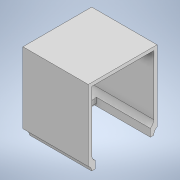
# Autodesk Inventor part: NEMA17_Shroud
Saved by Autodesk Inventor 2021 (Build 250183000, 183)
## iProperties
Created: 2021-10-06
Part Number: NEMA17_Shroud
Material: Generic
Document SubType Name: Modeling
Designer: Jorian Brusind
Density: 1 g/cm^3
Appearance: Default
Author: Jorian Brusind
Autodesk Inventor part; units mm, degrees
ref_plane "YZ Plane" through (0, 0, 0) normal (1, 0, 0) x (0, 1, 0)
ref_plane "XZ Plane" through (0, 0, 0) normal (0, 1, 0) x (-1, 0, 0)
ref_plane "XY Plane" through (0, 0, 0) normal (0, 0, 1) x (1, 0, 0)
sketch "Sketch1" plane through (0, 0, 0) normal (0, 1, 0) x (-1, 0, 0)
  line L0 (0, 0) -> (55, 0)
  line L1 (55, 0) -> (55, -55)
  line L2 (55, -55) -> (0, -55)
  line L3 (0, -58) -> (58, -58)
  line L4 (58, -58) -> (58, 3)
  line L5 (58, 3) -> (0, 3)
  line L6 (0, 3) -> (0, 0)
  line L7 (0, -55) -> (0, -58)
  dimension "d0" = 55
  dimension "d1" = 55
  dimension "d2" = 3
  constraints: 16 end point, 3 equal length, 2 perpendicular, 1 horizontal, 1 vertical, 2 other
  measures "d0" distance of L1.end L2.end
  measures "d1" distance of L0.end L1.end
  measures "d2" distance between parallel lines of L1 L4
extrude "Extrusion1" add sketch "Sketch1" along normal blind 60
sketch "Sketch2" plane through (0, 60, 0) normal (0, 1, 0) x (1, 0, 0)
  line L0 (-58, 58) -> (-58, -3) projected
  line L1 (0, 55) -> (0, 58) projected
  line L2 (-58, -3) -> (0, -3)
  line L3 (0, -3) -> (0, 58)
  line L4 (0, 58) -> (-58, 58)
  line L5 (-58, 58) -> (-58, -3)
  point P0 (0, 0)
  constraints: 8 end point, 2 parallel, 1 horizontal, 1 perpendicular
extrude "Extrusion2" add sketch "Sketch2" along normal blind 3
ref_plane "Work Plane1" through (0, -5, 0) normal (0, -1, 0) x (1, 0, 0)
sketch "Sketch3" plane through (0, -5, 0) normal (0, -1, 0) x (1, 0, 0)
  line L0 (-55, 0) -> (-55, -55) projected
  line L1 (-55, -55) -> (0, -55)
  line L2 (0, -55) -> (0, 0)
  line L3 (0, 0) -> (-55, 0)
  line L4 (-55, 0) -> (-55, -55)
  line L5 (-55, -27.5) -> (-48, -27.5)
  line L6 (-55, -27.5) -> (-48, -27.5) construction
  line L7 (-55, -55) -> (0, -55) projected
  line L8 (-27.5, -55) -> (-27.5, -52)
  line L9 (0, 0) -> (-55, 0) projected
  line L10 (-27.5, 0) -> (-27.5, -3)
  line L11 (-48, -27.5) -> (-48, -3)
  line L12 (-48, -3) -> (-27.5, -3)
  line L13 (-27.5, -52) -> (-48, -52)
  line L14 (-48, -52) -> (-48, -27.5)
  line L15 (-27.5, -52) -> (0, -52)
  line L16 (0, 3) -> (0, -58) projected
  line L17 (-27.5, -3) -> (0, -3)
  line L18 (0, -55) -> (0, -52)
  line L19 (0, -3) -> (0, 0)
  dimension "d8" = 7
  dimension "d9" = 0
  dimension "d10" = 3
  dimension "d11" = 3
  constraints: 32 end point, 5 point on line, 3 collinear, 3 horizontal, 3 midpoint, 3 parallel, 3 perpendicular, 3 vertical
  measures "d8" distance of L5.start L5.end
  measures "d9" distance between parallel lines of L5 L6
  measures "d10" distance of L8.start L8.end
  measures "d11" distance of L10.start L10.end
extrude "Extrusion3" add sketch "Sketch3" against normal blind 6 contours L3 L10 L12 L11 L5 L0 | L5 L14 L13 L8 L1 L0 | L3 L2 L17 L10 | L8 L15 L2 L1
fillet "Fillet5" radius 6 3 edges at (-27.5, 0, 0) (-55, 0, -27.5) (-27.5, 0, -55)
fillet "Fillet6" radius 6 3 edges at (-27.5, 1, 0) (-55, 1, -27.5) (-27.5, 1, -55)
fillet "Fillet7" radius 2 1 edges at (-48, -5, -27.5)
body "Solid1"
